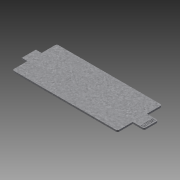
# Autodesk Inventor part: LogicPCB
Saved by Autodesk Inventor 2016 (Build 200138000, 138)
## iProperties
Created: 2015-06-09
Part Number: LogicPCB
Material: GFRC
Document SubType Name: Modeling
Designer: Yann
Density: 1.7 g/cm^3
Appearance: Flat - Polished Gray
Author: Yann
Autodesk Inventor part; units mm, degrees
ref_plane "YZ Plane" through (0, 0, 0) normal (1, 0, 0) x (0, 1, 0)
ref_plane "XZ Plane" through (0, 0, 0) normal (0, 1, 0) x (-1, 0, 0)
ref_plane "XY Plane" through (0, 0, 0) normal (0, 0, 1) x (1, 0, 0)
sketch "Sketch1" plane through (0, 0, 0) normal (0, 0, 1) x (1, 0, 0)
  line L0 (0, 39.0799) -> (0, -39.0799) construction
  line L1 (-102.2828, 0) -> (109.6971, 0) construction
  line L2 (0, 27.5) -> (63, 27.5)
  line L3 (65, 25.5) -> (65, 8.75)
  line L4 (65, 8.75) -> (77, 8.75)
  line L5 (79, 6.75) -> (79, 0)
  circle A0 centre (74, 6.75) radius 0.5
  circle A1 centre (75.5, 6.75) radius 0.5
  circle A2 centre (77, 6.75) radius 0.5
  circle A3 centre (74, 5.25) radius 0.5
  circle A4 centre (75.5, 5.25) radius 0.5
  circle A5 centre (77, 5.25) radius 0.5
  circle A6 centre (74, 3.75) radius 0.5
  circle A7 centre (75.5, 3.75) radius 0.5
  circle A8 centre (77, 3.75) radius 0.5
  circle A9 centre (74, 2.25) radius 0.5
  circle A10 centre (75.5, 2.25) radius 0.5
  circle A11 centre (77, 2.25) radius 0.5
  circle A12 centre (74, 0.75) radius 0.5
  circle A13 centre (75.5, 0.75) radius 0.5
  circle A14 centre (77, 0.75) radius 0.5
  circle A15 centre (74, -0.75) radius 0.5
  circle A16 centre (75.5, -0.75) radius 0.5
  circle A17 centre (77, -0.75) radius 0.5
  circle A18 centre (74, -2.25) radius 0.5
  circle A19 centre (75.5, -2.25) radius 0.5
  circle A20 centre (77, -2.25) radius 0.5
  circle A21 centre (74, -3.75) radius 0.5
  circle A22 centre (75.5, -3.75) radius 0.5
  circle A23 centre (77, -3.75) radius 0.5
  circle A24 centre (74, -5.25) radius 0.5
  circle A25 centre (75.5, -5.25) radius 0.5
  circle A26 centre (77, -5.25) radius 0.5
  circle A27 centre (74, -6.75) radius 0.5
  circle A28 centre (75.5, -6.75) radius 0.5
  circle A29 centre (77, -6.75) radius 0.5
  arc A30 (79, 6.75) -> (77, 8.75) centre (77, 6.75) ccw
  arc A31 (65, 25.5) -> (63, 27.5) centre (63, 25.5) ccw
  line L6 (0, -27.5) -> (63, -27.5)
  line L7 (65, -25.5) -> (65, -8.75)
  line L8 (65, -8.75) -> (77, -8.75)
  line L9 (79, -6.75) -> (79, 0)
  arc A32 (77, -8.75) -> (79, -6.75) centre (77, -6.75) ccw
  arc A33 (63, -27.5) -> (65, -25.5) centre (63, -25.5) ccw
  line L10 (0, 27.5) -> (-63, 27.5)
  line L11 (-65, 25.5) -> (-65, 8.75)
  arc A34 (-63, 27.5) -> (-65, 25.5) centre (-63, 25.5) ccw
  line L12 (0, -27.5) -> (-63, -27.5)
  line L13 (-65, -25.5) -> (-65, -8.75)
  arc A35 (-65, -25.5) -> (-63, -27.5) centre (-63, -25.5) ccw
  line L14 (-65, 8.75) -> (-72, 8.75)
  line L15 (-72, 8.75) -> (-72, -8.75)
  line L16 (-65, -8.75) -> (-72, -8.75)
  line L17 (72, 8.75) -> (72, -8.75) construction
  point P0 (0, 0)
  dimension "d0" = 27.5
  dimension "d2" = 1
  dimension "d5" = 1.5
  dimension "d8" = 1.5
  dimension "d11" = 2
  dimension "d12" = 2
  dimension "d13" = 2
  dimension "d16" = 2
  dimension "d19" = 65
  dimension "d20" = 2
  dimension "d21" = 7
  dimension "d22" = 7
  constraints: 36 centre point, 32 end point, 17 symmetric about line, 12 point on circle, 5 perpendicular, 4 point on line, 4 tangent, 2 horizontal, 1 vertical, 62 other
  measures "d0" distance between parallel lines of L1 L2
  measures "d2" diameter of A0
  measures "d5" distance of A0.centre A1.centre
  measures "d8" distance of A0.centre A3.centre
  measures "d11" distance from line of L5 A17.centre
  measures "d12" distance from line of L4 A2.centre
  measures "d13" radius of A30
  measures "d16" radius of A31
  measures "d19" distance between parallel lines of L7 L0
  measures "d20" distance from line of A18.centre L17
  measures "d21" distance between parallel lines of L7 L17
  measures "d22" distance between parallel lines of L13 L15
extrude "Extrusion1" add sketch "Sketch1" along normal blind 2
equation "\"d0\" = 0.5 * LogicPCB_Width"
equation "\"d12\" = d11"
equation "\"d19\" = 0.5 * PowerPCB_Length"
equation "\"d21\" = Interface_Thickness"
equation "\"d22\" = Interface_Thickness"
equation "\"d17\" = LogicPCB_Thickness"
equation "\"LogicPCB_Width\" = 55"
equation "\"LogicPCB_Thickness\" = 2"
equation "\"Heatsink_Thickness\" = 7"
equation "\"Heatsink_Width\" = 65"
equation "\"Cover_Thickness\" = 2"
equation "\"PowerPCB_Minus_Height\" = 1.2"
equation "\"Interface_Thickness\" = 7"
equation "\"PowerPCB_Thickness\" = 3"
equation "\"PowerPCB_Plus_Height\" = 8"
equation "\"LogicPCB_Plus_Height\" = 8"
equation "\"HostPCB_Thickness\" = 1.2"
equation "\"HostPCB_Plus_Height\" = 8"
equation "\"PowerPCB_Length\" = 130"
body "Solid1"
